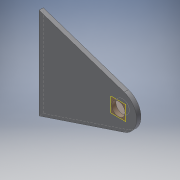
# Autodesk Inventor part: left stand
Saved by Autodesk Inventor 2019 (Build 230136000, 136)
## iProperties
Created: 2022-03-28
Part Number: left stand
Material: Generic
Document SubType Name: Modeling
Designer: Ian
Density: 1 g/cm^3
Appearance: Default
Author: Ian
Autodesk Inventor part; units mm, degrees
ref_plane "YZ Plane" through (0, 0, 0) normal (1, 0, 0) x (0, 1, 0)
ref_plane "XZ Plane" through (0, 0, 0) normal (0, 1, 0) x (-1, 0, 0)
ref_plane "XY Plane" through (0, 0, 0) normal (0, 0, 1) x (1, 0, 0)
ref_plane "Work Plane1" through (0, 0, 0) normal (0, 0, 1) x (1, 0, 0)
sketch "Sketch1" plane through (0, 0, 0) normal (0, 0, 1) x (1, 0, 0)
  line L0 (0, 0) -> (-130, 0)
  line L1 (-130, 0) -> (-130, -75)
  line L2 (-130, 0) -> (-130, 75)
  circle A0 centre (0, 0) radius 11 projected
  circle A1 centre (0, 0) radius 30
  line L3 (9.4949, 28.4578) -> (-130, 75)
  line L4 (9.4949, -28.4578) -> (-130, -75)
  dimension "d2" = 60
  dimension "d3" = 150
  dimension "d4" = 130
  constraints: 10 end point, 2 point on circle, 2 tangent, 1 centre point, 1 coincident, 1 collinear, 1 horizontal, 1 perpendicular, 1 vertical
  measures "d2" diameter of A1
  measures "d3" distance of L2.end L1.end
  measures "d4" distance of L0.start L0.end
extrude "Extrusion1" add sketch "Sketch1" against normal blind 7
body "Solid1"
